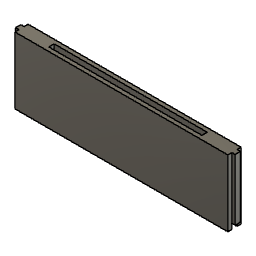
wall_ (Autodesk Fusion 360 design; units mm, degrees)
Autodesk Fusion 360 part; units mm, degrees
sketch "Esquisse1" plane through (0, 0, 0) normal (0, 1, 0) x (1, 0, 0)
  line L0 (0, 0) -> (-160, 0)
  line L1 (-160, 0) -> (-160, 3)
  line L2 (-160, 3) -> (0, 3)
  line L3 (0, 3) -> (0, 0)
  line L4 (0, 7) -> (-160, 7)
  line L5 (-160, 7) -> (-160, 10)
  line L6 (-160, 10) -> (0, 10)
  line L7 (0, 10) -> (0, 7)
  line L8 (-137.5, 3) -> (-162.5, 3)
  line L9 (-162.5, 3) -> (-162.5, 7)
  line L10 (-162.5, 7) -> (-137.5, 7)
  line L11 (-137.5, 7) -> (-137.5, 3)
  line L12 (-22.5, 7) -> (2.5, 7)
  line L13 (2.5, 7) -> (2.5, 3)
  line L14 (2.5, 3) -> (-22.5, 3)
  line L15 (-22.5, 3) -> (-22.5, 7)
  dimension "d1" = 160
  dimension "d2" = 3
  dimension "d3" = 160
  dimension "d4" = 3
  dimension "d5" = 4
  dimension "d6" = 25
  dimension "d7" = 2.5
  dimension "d8" = 4
  dimension "d9" = 4
  dimension "d10" = 25
  dimension "d11" = 2.5
  constraint horizontal L0
  constraint vertical L1
  constraint horizontal L2
  constraint vertical L3
  constraint coincident L0.start L3.end
  constraint horizontal L4
  constraint vertical L5
  constraint horizontal L6
  constraint vertical L7
  constraint horizontal L8
  constraint vertical L9
  constraint horizontal L10
  constraint vertical L11
  constraint coincident L2 L8.start
  constraint horizontal L12
  constraint vertical L13
  constraint horizontal L14
  constraint vertical L15
  constraint coincident L4 L12.start
  measures "d1" distance of L0.start L0.end
  measures "d2" distance of L0.start L2.end
  measures "d3" distance of L5.end L6.end
  measures "d4" distance of L4.start L6.end
  measures "d5" distance of L2.end L4.start
  measures "d6" distance of L8.start L8.end
  measures "d7" distance of L1.end L8.end
  measures "d8" distance of L8.end L9.end
  measures "d9" distance of L12.end L13.end
  measures "d10" distance of L12.start L12.end
  measures "d11" distance of L2.end L13.end
extrude "Extrusion1" add sketch "Esquisse1" along normal blind 50 contours L0 L1 L2 L3 L8 L14 | L2 L4 L12 L13 L14 L15 | L2 L4 L8 L9 L10 L11 | L4 L5 L6 L7 L10 L12
sketch "Esquisse2" plane through (0, 0, 0) normal (0, -1, 0) x (1, 0, 0)
  line L0 (-22.5, -3) -> (-22.5, -7)
  line L1 (-22.5, -7) -> (-137.5, -7)
  line L2 (-137.5, -7) -> (-137.5, -3)
  line L3 (-137.5, -3) -> (-22.5, -3)
  line L4 (2.5, -7) -> (2.5, -3)
  line L5 (2.5, -3) -> (0, -3)
  line L6 (0, -3) -> (0, 0)
  line L7 (0, 0) -> (-160, 0)
  line L8 (-160, 0) -> (-160, -3)
  line L9 (-160, -3) -> (-162.5, -3)
  line L10 (-162.5, -3) -> (-162.5, -7)
  line L11 (-162.5, -7) -> (-160, -7)
  line L12 (-160, -7) -> (-160, -10)
  line L13 (-160, -10) -> (0, -10)
  line L14 (0, -10) -> (0, -7)
  line L15 (0, -7) -> (2.5, -7)
  line L16 (-22.5, -3) -> (2.5, -3)
  line L17 (2.5, -3) -> (2.5, -7)
  line L18 (2.5, -7) -> (-22.5, -7)
  line L19 (-22.5, -7) -> (-22.5, -3)
  line L20 (-137.5, -7) -> (-162.5, -7)
  line L21 (-162.5, -7) -> (-162.5, -3)
  line L22 (-162.5, -3) -> (-137.5, -3)
  line L23 (-137.5, -3) -> (-137.5, -7)
  constraint horizontal L16
  constraint vertical L17
  constraint horizontal L18
  constraint vertical L19
  constraint coincident L4.start L15.end
  constraint coincident L0.start L3.end
  constraint horizontal L20
  constraint vertical L21
  constraint horizontal L22
  constraint vertical L23
  constraint coincident L9.end L10.start
  constraint coincident L1.end L2.start
extrude "Extrusion2" cut sketch "Esquisse2" against normal blind 4 contours L0 L4 L5 L15 L16 L17 L18 L19 | L2 L9 L10 L11 L20 L21 L22 L23
